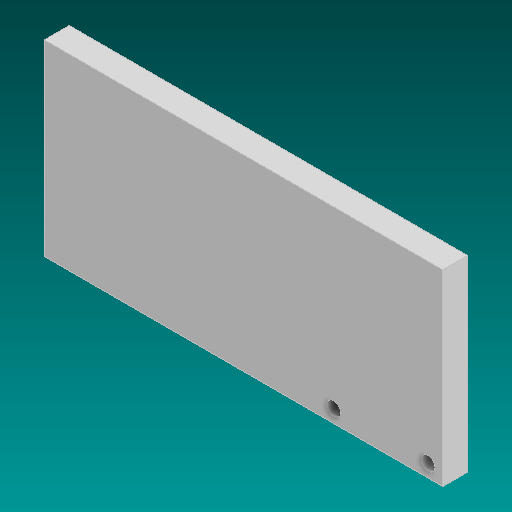
# Autodesk Inventor part: Part19
Saved by Autodesk Inventor 2020 (Build 240168000, 168)
## iProperties
Created: 2022-11-16
Part Number: Part19
Material: 一般
Document SubType Name: Modeling
Designer: Administrator
Density: 1 g/cm^3
Appearance: 既定
Author: Administrator
Autodesk Inventor part; units mm, degrees
ref_plane "YZ Plane" through (0, 0, 0) normal (1, 0, 0) x (0, 1, 0)
ref_plane "XZ Plane" through (0, 0, 0) normal (0, 1, 0) x (-1, 0, 0)
ref_plane "XY Plane" through (0, 0, 0) normal (0, 0, 1) x (1, 0, 0)
sketch "スケッチ1" plane through (0, 0, 0) normal (0, 0, 1) x (1, 0, 0)
  line L0 (50, -5) -> (-110.2322, -5)
  line L1 (-110.2322, -5) -> (-110.2322, 70.4763)
  line L2 (-110.2322, 70.4763) -> (50, 70.4763)
  line L3 (50, 70.4763) -> (50, -5)
  circle A0 centre (44, 0) radius 2.75 projected
  circle A1 centre (6, 0) radius 2.75 projected
  point P0 (0, 0)
  constraints: 8 end point, 2 parallel, 1 horizontal, 1 perpendicular, 1 other
extrude "押し出し1" add sketch "スケッチ1" along normal blind 10
